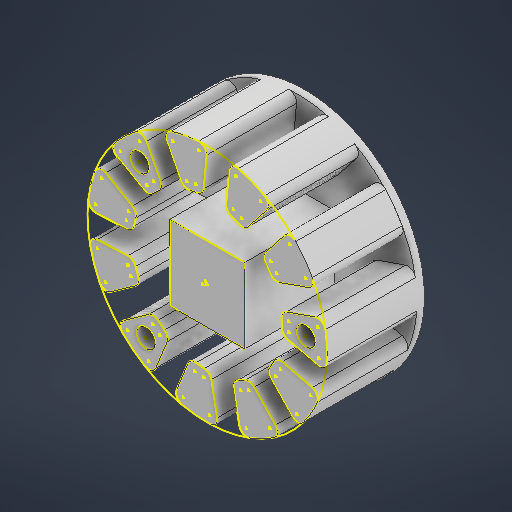
# Autodesk Inventor part: новая сиська 5-26
Saved by Autodesk Inventor 2025 (Build 290162000, 162)
## iProperties
Created: 2025-10-01
Part Number: новая сиська 5-26
Material: Типовые
Document SubType Name: Modeling
Designer: GameHD
Density: 1 g/cm^3
Appearance: По умолчанию
Author: GameHD
Autodesk Inventor part; units mm, degrees
ref_plane "YZ Plane" through (0, 0, 0) normal (1, 0, 0) x (0, 1, 0)
ref_plane "XZ Plane" through (0, 0, 0) normal (0, 1, 0) x (-1, 0, 0)
ref_plane "XY Plane" through (0, 0, 0) normal (0, 0, 1) x (1, 0, 0)
sketch "Эскиз1" plane through (0, 0, 0) normal (0, 0, 1) x (1, 0, 0)
  arc A0 (22.5563, 14.1182) -> (20.9448, 16.3602) centre (1.564, 0.7293) ccw
  arc A1 (20.9188, 19.4663) -> (20.9448, 16.3602) centre (22.8907, 17.9297) ccw
  line L0 (20.9188, 19.4663) -> (27.2495, 27.5902)
  arc A2 (31.0653, 27.7418) -> (27.2495, 27.5902) centre (29.2214, 26.0536) ccw
  arc A3 (36.5698, 20.0838) -> (31.0653, 27.7418) centre (1.564, 0.7293) ccw
  arc A4 (35.2101, 16.5153) -> (36.5698, 20.0838) centre (34.382, 18.8741) ccw
  line L1 (35.2101, 16.5153) -> (25.4922, 13.1036)
  arc A5 (22.5563, 14.1182) -> (25.4922, 13.1036) centre (24.6641, 15.4625) ccw
  line L2 (-22.3857, -11.7684) -> (-30.7753, -17.7426)
  arc A6 (-34.475, -16.7967) -> (-30.7753, -17.7426) centre (-32.2254, -15.7062) ccw
  arc A7 (-37.5597, -7.8842) -> (-34.475, -16.7967) centre (1.5191, 0.651) ccw
  arc A8 (-35.2362, -4.8536) -> (-37.5597, -7.8842) centre (-35.1172, -7.3508) ccw
  line L3 (-35.2362, -4.8536) -> (-24.9486, -4.3636)
  arc A9 (-22.4254, -6.1753) -> (-24.9486, -4.3636) centre (-24.8296, -6.8607) ccw
  arc A10 (-22.4254, -6.1753) -> (-21.5223, -8.7846) centre (1.5191, 0.651) ccw
  arc A11 (-22.3857, -11.7684) -> (-21.5223, -8.7846) centre (-23.8358, -9.732) ccw
  line L4 (-11.8764, -22.7208) -> (-15.7043, -32.2823)
  arc A12 (-19.3282, -33.4868) -> (-15.7043, -32.2823) centre (-18.0252, -31.3532) ccw
  arc A13 (-26.7415, -27.6569) -> (-19.3282, -33.4868) centre (1.5191, 0.651) ccw
  arc A14 (-26.4254, -23.8512) -> (-26.7415, -27.6569) centre (-24.9752, -25.8876) ccw
  line L5 (-26.4254, -23.8512) -> (-18.0358, -17.877)
  arc A15 (-14.9337, -18.037) -> (-18.0358, -17.877) centre (-16.5857, -19.9134) ccw
  arc A16 (-14.9337, -18.037) -> (-12.7633, -19.7438) centre (1.5191, 0.651) ccw
  arc A17 (-11.8764, -22.7208) -> (-12.7633, -19.7438) centre (-14.1973, -21.7916) ccw
  line L6 (-19.7085, 17.2364) -> (-28.6279, 22.386)
  arc A18 (-29.3044, 26.1444) -> (-28.6279, 22.386) centre (-27.3779, 24.5511) ccw
  arc A19 (-22.4788, 32.6526) -> (-29.3044, 26.1444) centre (1.5191, 0.651) ccw
  arc A20 (-18.7568, 31.7981) -> (-22.4788, 32.6526) centre (-20.9789, 30.6525) ccw
  line L7 (-18.7568, 31.7981) -> (-14.0374, 22.6437)
  arc A21 (-14.6373, 19.5959) -> (-14.0374, 22.6437) centre (-16.2595, 21.4982) ccw
  arc A22 (-14.6373, 19.5959) -> (-16.6356, 17.6905) centre (1.5191, 0.651) ccw
  arc A23 (-19.7085, 17.2364) -> (-16.6356, 17.6905) centre (-18.4585, 19.4014) ccw
  line L8 (26.5594, -9.282) -> (36.5684, -11.7101)
  arc A24 (38.2763, -15.1257) -> (36.5684, -11.7101) centre (35.979, -14.1397) ccw
  arc A25 (33.5608, -23.2933) -> (38.2763, -15.1257) centre (1.5191, 0.651) ccw
  arc A26 (29.7488, -23.522) -> (33.5608, -23.2933) centre (31.5582, -21.7968) ccw
  line L9 (29.7488, -23.522) -> (22.6415, -16.068)
  arc A27 (22.3584, -12.9747) -> (22.6415, -16.068) centre (24.4508, -14.3428) ccw
  arc A28 (22.3584, -12.9747) -> (23.739, -10.5835) centre (1.5191, 0.651) ccw
  arc A29 (26.5594, -9.282) -> (23.739, -10.5835) centre (25.97, -11.7115) ccw
  line L10 (27.9545, 5.8327) -> (37.6874, 9.2013)
  arc A30 (40.9708, 7.2513) -> (37.6874, 9.2013) centre (38.5051, 6.8388) ccw
  arc A31 (41.4196, -2.1692) -> (40.9708, 7.2513) centre (1.5191, 0.651) ccw
  arc A32 (38.3364, -4.4224) -> (41.4196, -2.1692) centre (38.9258, -1.9929) ccw
  line L11 (38.3364, -4.4224) -> (28.3274, -1.9943)
  arc A33 (26.4169, 0.4549) -> (28.3274, -1.9943) centre (28.9168, 0.4352) ccw
  arc A34 (26.4169, 0.4549) -> (26.2855, 3.2129) centre (1.5191, 0.651) ccw
  arc A35 (27.9545, 5.8327) -> (26.2855, 3.2129) centre (28.7722, 3.4702) ccw
  line L12 (-7.372, 26.08) -> (-12.0914, 35.2344)
  arc A36 (-10.6285, 38.7619) -> (-12.0914, 35.2344) centre (-9.8693, 36.3799) ccw
  arc A37 (-1.3678, 40.5467) -> (-10.6285, 38.7619) centre (1.5191, 0.651) ccw
  arc A38 (1.3013, 37.8156) -> (-1.3678, 40.5467) centre (-1.1874, 38.0532) ccw
  line L13 (1.3013, 37.8156) -> (0.3223, 27.5629)
  arc A39 (-1.8301, 25.3233) -> (0.3223, 27.5629) centre (-2.1664, 27.8006) ccw
  arc A40 (-1.8301, 25.3233) -> (-4.5414, 24.8007) centre (1.5191, 0.651) ccw
  arc A41 (-7.372, 26.08) -> (-4.5414, 24.8007) centre (-5.1499, 27.2256) ccw
  line L14 (2.8858, -26.2528) -> (4.835, -36.3659)
  arc A42 (2.4376, -39.3384) -> (4.835, -36.3659) centre (2.3802, -36.8391) ccw
  arc A43 (-6.9508, -38.4419) -> (2.4376, -39.3384) centre (1.5191, 0.651) ccw
  arc A44 (-8.7424, -35.0695) -> (-6.9508, -38.4419) centre (-6.4215, -35.9986) ccw
  line L15 (-8.7424, -35.0695) -> (-4.9145, -25.5079)
  arc A45 (-2.2183, -23.9654) -> (-4.9145, -25.5079) centre (-2.5936, -26.4371) ccw
  arc A46 (-2.2183, -23.9654) -> (0.5303, -24.2279) centre (1.5191, 0.651) ccw
  arc A47 (2.8858, -26.2528) -> (0.5303, -24.2279) centre (0.431, -26.7259) ccw
  line L16 (-25.3054, 3.127) -> (-35.593, 2.637)
  arc A48 (-38.194, 5.433) -> (-35.593, 2.637) centre (-35.712, 5.1341) ccw
  arc A49 (-35.9706, 14.5983) -> (-38.194, 5.433) centre (1.5191, 0.651) ccw
  arc A50 (-32.3775, 15.8916) -> (-35.9706, 14.5983) centre (-33.6275, 13.7266) ccw
  line L17 (-32.3775, 15.8916) -> (-23.458, 10.742)
  arc A51 (-22.3149, 7.8537) -> (-23.458, 10.742) centre (-24.708, 8.5769) ccw
  arc A52 (-22.3149, 7.8537) -> (-22.9659, 5.1704) centre (1.5191, 0.651) ccw
  arc A53 (-25.3054, 3.127) -> (-22.9659, 5.1704) centre (-25.4243, 5.6242) ccw
  line L18 (17.2148, -21.2437) -> (24.3215, -28.6969)
  arc A54 (23.9117, -32.4937) -> (24.3215, -28.6969) centre (22.5122, -30.4221) ccw
  arc A55 (15.529, -36.8153) -> (23.9117, -32.4937) centre (1.5191, 0.651) ccw
  arc A56 (12.1985, -34.9467) -> (15.529, -36.8153) centre (14.6534, -34.4736) ccw
  line L19 (12.1985, -34.9467) -> (10.2513, -24.8433)
  arc A57 (11.676, -22.0923) -> (10.2513, -24.8433) centre (12.7061, -24.3702) ccw
  arc A58 (11.676, -22.0923) -> (14.1352, -20.8156) centre (1.1306, 1.228) ccw
  arc A59 (17.2148, -21.2437) -> (14.1352, -20.8156) centre (15.4055, -22.9689) ccw
  line L20 (7.7874, 26.8501) -> (8.7664, 37.1028)
  arc A60 (11.9042, 39.2794) -> (8.7664, 37.1028) centre (11.2551, 36.8651) ccw
  arc A61 (20.6597, 35.7742) -> (11.9042, 39.2794) centre (1.5191, 0.651) ccw
  arc A62 (21.4285, 32.0336) -> (20.6597, 35.7742) centre (19.4634, 33.579) ccw
  line L21 (21.4285, 32.0336) -> (15.0619, 23.9378)
  arc A63 (12.0404, 23.2174) -> (15.0619, 23.9378) centre (13.0968, 25.4832) ccw
  arc A64 (12.0404, 23.2174) -> (9.477, 24.2436) centre (1.5191, 0.651) ccw
  arc A65 (7.7874, 26.8501) -> (9.477, 24.2436) centre (10.2761, 26.6125) ccw
  circle A66 centre (1.5191, 0.651) radius 50
  line L22 (19.1721, 10.843) -> (19.1721, -9.5409)
  line L23 (19.1721, -9.5409) -> (1.5191, -19.7329)
  line L24 (1.5191, -19.7329) -> (-16.1339, -9.5409)
  line L25 (-16.1339, -9.5409) -> (-16.1339, 10.843)
  line L26 (-16.1339, 10.843) -> (1.5191, 21.035)
  line L27 (1.5191, 21.035) -> (19.1721, 10.843)
  point P0 (0, 0)
  point P1 (1.5191, 0.651)
  dimension "d9" = 100
  constraints: 132 point on circle, 67 centre point, 56 end point
  measures "d9" diameter of A66
extrude "Выдавливание1" add sketch "Эскиз1" along normal blind 30 contours A0 A1 L0 A2 A3 A4 L1 A5 | L2 A6 A7 A8 L3 A9 A10 A11 | L4 A12 A13 A14 L5 A15 A16 A17 | L6 A18 A19 A20 L7 A21 A22 A23 | L8 A24 A25 A26 L9 A27 A28 A29 | L10 A30 A31 A32 L11 A33 A34 A35 | L12 A36 A37 A38 L13 A39 A40 A41 | L14 A42 A43 A44 L15 A45 A46 A47 | L16 A48 A49 A50 L17 A51 A52 A53 | L18 A54 A55 A56 L19 A57 A58 A59 | L20 A60 A61 A62 L21 A63 A64 A65 | L22 L23 L24 L25 L26 L27
sketch "Эскиз2" plane through (0, 0, 0) normal (0, 0, -1) x (-1, 0, 0)
  line L0 (-19.1721, 10.843) -> (-1.5191, 21.035) projected
  line L1 (-19.1721, -9.5409) -> (-19.1721, 10.843) projected
  line L2 (-1.5191, -19.7329) -> (-19.1721, -9.5409) projected
  line L3 (16.1339, -9.5409) -> (-1.5191, -19.7329) projected
  line L4 (16.1339, 10.843) -> (16.1339, -9.5409) projected
  line L5 (-1.5191, 21.035) -> (16.1339, 10.843) projected
  arc A0 (-11.9042, 39.2794) -> (-20.6597, 35.7742) centre (-1.5191, 0.651) ccw projected
  circle A1 centre (-1.5191, 0.651) radius 40
  point P0 (0, 0)
  dimension "d2" = 80
  constraints: 1 centre point, 1 coincident
  measures "d2" diameter of A1
extrude "Выдавливание2" add sketch "Эскиз2" along normal blind 2.5 contours L0 L5 L4 L3 L2 L1 | A1 A0
sketch "Эскиз3" plane through (0, 0, 30) normal (0, 0, 1) x (1, 0, 0)
  line L0 (19.1721, 10.843) -> (1.5191, 21.035) projected
  line L1 (1.5191, 21.035) -> (-16.1339, 10.843) projected
  line L2 (-16.1339, 10.843) -> (-16.1339, -9.5409) projected
  line L3 (-16.1339, -9.5409) -> (1.5191, -19.7329) projected
  line L4 (1.5191, -19.7329) -> (19.1721, -9.5409) projected
  line L5 (19.1721, -9.5409) -> (19.1721, 10.843) projected
  arc A0 (-22.4788, 32.6526) -> (-29.3044, 26.1444) centre (1.5191, 0.651) ccw projected
  line L6 (14.0191, -11.849) -> (-10.9809, -11.849)
  line L7 (-10.9809, -11.849) -> (-10.9809, 13.151)
  line L8 (-10.9809, 13.151) -> (14.0191, 13.151)
  line L9 (14.0191, 13.151) -> (14.0191, -11.849)
  line L10 (14.0191, -11.849) -> (-10.9809, 13.151) construction
  line L11 (-10.9809, -11.849) -> (14.0191, 13.151) construction
  point P0 (0, 0)
  dimension "d5" = 25
  dimension "d6" = 25
  constraints: 12 end point, 2 midpoint, 2 parallel, 1 horizontal, 1 perpendicular
  measures "d5" distance of L7.end L8.end
  measures "d6" distance of L6.end L7.end
extrude "Выдавливание3" cut sketch "Эскиз3" against normal up to surface (30 mm away)
sketch "Эскиз6" plane through (0, 0, 30) normal (0, 0, 1) x (1, 0, 0)
  circle A0 centre (34.4254, 2.0527) radius 3.1 projected
  circle A1 centre (-21.0893, 24.6021) radius 3.1 projected
  circle A2 centre (-18.9706, -25.1358) radius 3.1 projected
  point P0 (0, 0)
extrude "Выдавливание5" cut sketch "Эскиз6" against normal through all
sketch "Эскиз7" plane through (0, 0, 30) normal (0, 0, 1) x (1, 0, 0)
  line L0 (-10.9809, -11.849) -> (-10.9809, 13.151) projected
  line L1 (-10.9809, 13.151) -> (14.0191, 13.151) projected
  line L2 (14.0191, 13.151) -> (14.0191, -11.849) projected
  line L3 (14.0191, -11.849) -> (-10.9809, -11.849) projected
  arc A0 (21.4285, 32.0336) -> (20.6597, 35.7742) centre (19.4634, 33.579) ccw projected
  line L4 (15.0619, 23.9378) -> (21.4285, 32.0336) projected
  arc A1 (12.0404, 23.2174) -> (15.0619, 23.9378) centre (13.0968, 25.4832) ccw projected
  arc A2 (12.0404, 23.2174) -> (9.477, 24.2436) centre (1.5191, 0.651) ccw projected
  arc A3 (7.7874, 26.8501) -> (9.477, 24.2436) centre (10.2761, 26.6125) ccw projected
  line L5 (8.7664, 37.1028) -> (7.7874, 26.8501) projected
  arc A4 (11.9042, 39.2794) -> (8.7664, 37.1028) centre (11.2551, 36.8651) ccw projected
  arc A5 (11.9042, 39.2794) -> (-1.3678, 40.5467) centre (1.5191, 0.651) ccw projected
  arc A6 (1.3013, 37.8156) -> (-1.3678, 40.5467) centre (-1.1874, 38.0532) ccw projected
  line L6 (0.3223, 27.5629) -> (1.3013, 37.8156) projected
  arc A7 (-1.8301, 25.3233) -> (0.3223, 27.5629) centre (-2.1664, 27.8006) ccw projected
  arc A8 (-1.8301, 25.3233) -> (-4.5414, 24.8007) centre (1.5191, 0.651) ccw projected
  arc A9 (-7.372, 26.08) -> (-4.5414, 24.8007) centre (-5.1499, 27.2256) ccw projected
  line L7 (-12.0914, 35.2344) -> (-7.372, 26.08) projected
  arc A10 (-10.6285, 38.7619) -> (-12.0914, 35.2344) centre (-9.8693, 36.3799) ccw projected
  arc A11 (-10.6285, 38.7619) -> (-22.4788, 32.6526) centre (1.5191, 0.651) ccw projected
  arc A12 (-18.7568, 31.7981) -> (-22.4788, 32.6526) centre (-20.9789, 30.6525) ccw projected
  line L8 (-14.0374, 22.6437) -> (-18.7568, 31.7981) projected
  arc A13 (-14.6373, 19.5959) -> (-14.0374, 22.6437) centre (-16.2595, 21.4982) ccw projected
  arc A14 (-14.6373, 19.5959) -> (-16.6356, 17.6905) centre (1.5191, 0.651) ccw projected
  arc A15 (-19.7085, 17.2364) -> (-16.6356, 17.6905) centre (-18.4585, 19.4014) ccw projected
  line L9 (-28.6279, 22.386) -> (-19.7085, 17.2364) projected
  arc A16 (-29.3044, 26.1444) -> (-28.6279, 22.386) centre (-27.3779, 24.5511) ccw projected
  arc A17 (-29.3044, 26.1444) -> (-35.9706, 14.5983) centre (1.5191, 0.651) ccw projected
  arc A18 (-32.3775, 15.8916) -> (-35.9706, 14.5983) centre (-33.6275, 13.7266) ccw projected
  line L10 (-23.458, 10.742) -> (-32.3775, 15.8916) projected
  arc A19 (-22.3149, 7.8537) -> (-23.458, 10.742) centre (-24.708, 8.5769) ccw projected
  arc A20 (-22.3149, 7.8537) -> (-22.9659, 5.1704) centre (1.5191, 0.651) ccw projected
  arc A21 (-25.3054, 3.127) -> (-22.9659, 5.1704) centre (-25.4243, 5.6242) ccw projected
  line L11 (-35.593, 2.637) -> (-25.3054, 3.127) projected
  arc A22 (-38.194, 5.433) -> (-35.593, 2.637) centre (-35.712, 5.1341) ccw projected
  arc A23 (-38.194, 5.433) -> (-37.5597, -7.8842) centre (1.5191, 0.651) ccw projected
  arc A24 (-35.2362, -4.8536) -> (-37.5597, -7.8842) centre (-35.1172, -7.3508) ccw projected
  line L12 (-24.9486, -4.3636) -> (-35.2362, -4.8536) projected
  arc A25 (-22.4254, -6.1753) -> (-24.9486, -4.3636) centre (-24.8296, -6.8607) ccw projected
  arc A26 (-22.4254, -6.1753) -> (-21.5223, -8.7846) centre (1.5191, 0.651) ccw projected
  arc A27 (-22.3857, -11.7684) -> (-21.5223, -8.7846) centre (-23.8358, -9.732) ccw projected
  line L13 (-30.7753, -17.7426) -> (-22.3857, -11.7684) projected
  arc A28 (-34.475, -16.7967) -> (-30.7753, -17.7426) centre (-32.2254, -15.7062) ccw projected
  arc A29 (-34.475, -16.7967) -> (-26.7415, -27.6569) centre (1.5191, 0.651) ccw projected
  arc A30 (-26.4254, -23.8512) -> (-26.7415, -27.6569) centre (-24.9752, -25.8876) ccw projected
  line L14 (-18.0358, -17.877) -> (-26.4254, -23.8512) projected
  arc A31 (-14.9337, -18.037) -> (-18.0358, -17.877) centre (-16.5857, -19.9134) ccw projected
  arc A32 (-14.9337, -18.037) -> (-12.7633, -19.7438) centre (1.5191, 0.651) ccw projected
  arc A33 (-11.8764, -22.7208) -> (-12.7633, -19.7438) centre (-14.1973, -21.7916) ccw projected
  line L15 (-15.7043, -32.2823) -> (-11.8764, -22.7208) projected
  arc A34 (-19.3282, -33.4868) -> (-15.7043, -32.2823) centre (-18.0252, -31.3532) ccw projected
  arc A35 (-19.3282, -33.4868) -> (-6.9508, -38.4419) centre (1.5191, 0.651) ccw projected
  arc A36 (-8.7424, -35.0695) -> (-6.9508, -38.4419) centre (-6.4215, -35.9986) ccw projected
  line L16 (-4.9145, -25.5079) -> (-8.7424, -35.0695) projected
  arc A37 (-2.2183, -23.9654) -> (-4.9145, -25.5079) centre (-2.5936, -26.4371) ccw projected
  arc A38 (-2.2183, -23.9654) -> (0.5303, -24.2279) centre (1.5191, 0.651) ccw projected
  arc A39 (2.8858, -26.2528) -> (0.5303, -24.2279) centre (0.431, -26.7259) ccw projected
  line L17 (4.835, -36.3659) -> (2.8858, -26.2528) projected
  arc A40 (2.4376, -39.3384) -> (4.835, -36.3659) centre (2.3802, -36.8391) ccw projected
  arc A41 (2.4376, -39.3384) -> (15.529, -36.8153) centre (1.5191, 0.651) ccw projected
  arc A42 (12.1985, -34.9467) -> (15.529, -36.8153) centre (14.6534, -34.4736) ccw projected
  line L18 (10.2513, -24.8433) -> (12.1985, -34.9467) projected
  arc A43 (11.676, -22.0923) -> (10.2513, -24.8433) centre (12.7061, -24.3702) ccw projected
  arc A44 (11.676, -22.0923) -> (14.1352, -20.8156) centre (1.1306, 1.228) ccw projected
  arc A45 (17.2148, -21.2437) -> (14.1352, -20.8156) centre (15.4055, -22.9689) ccw projected
  line L19 (24.3215, -28.6969) -> (17.2148, -21.2437) projected
  arc A46 (23.9117, -32.4937) -> (24.3215, -28.6969) centre (22.5122, -30.4221) ccw projected
  arc A47 (23.9117, -32.4937) -> (33.5608, -23.2933) centre (1.5191, 0.651) ccw projected
  arc A48 (29.7488, -23.522) -> (33.5608, -23.2933) centre (31.5582, -21.7968) ccw projected
  line L20 (22.6415, -16.068) -> (29.7488, -23.522) projected
  arc A49 (22.3584, -12.9747) -> (22.6415, -16.068) centre (24.4508, -14.3428) ccw projected
  arc A50 (22.3584, -12.9747) -> (23.739, -10.5835) centre (1.5191, 0.651) ccw projected
  arc A51 (26.5594, -9.282) -> (23.739, -10.5835) centre (25.97, -11.7115) ccw projected
  line L21 (36.5684, -11.7101) -> (26.5594, -9.282) projected
  arc A52 (38.2763, -15.1257) -> (36.5684, -11.7101) centre (35.979, -14.1397) ccw projected
  arc A53 (38.2763, -15.1257) -> (41.4196, -2.1692) centre (1.5191, 0.651) ccw projected
  arc A54 (38.3364, -4.4224) -> (41.4196, -2.1692) centre (38.9258, -1.9929) ccw projected
  line L22 (28.3274, -1.9943) -> (38.3364, -4.4224) projected
  arc A55 (26.4169, 0.4549) -> (28.3274, -1.9943) centre (28.9168, 0.4352) ccw projected
  arc A56 (26.4169, 0.4549) -> (26.2855, 3.2129) centre (1.5191, 0.651) ccw projected
  arc A57 (27.9545, 5.8327) -> (26.2855, 3.2129) centre (28.7722, 3.4702) ccw projected
  line L23 (37.6874, 9.2013) -> (27.9545, 5.8327) projected
  arc A58 (40.9708, 7.2513) -> (37.6874, 9.2013) centre (38.5051, 6.8388) ccw projected
  arc A59 (40.9708, 7.2513) -> (36.8048, 19.4902) centre (1.5191, 0.651) ccw projected
  arc A60 (35.2101, 16.5153) -> (36.8048, 19.4902) centre (34.382, 18.8741) ccw projected
  line L24 (25.4922, 13.1036) -> (35.2101, 16.5153) projected
  arc A61 (22.5563, 14.1182) -> (25.4922, 13.1036) centre (24.6641, 15.4625) ccw projected
  arc A62 (22.5563, 14.1182) -> (20.9448, 16.3602) centre (1.564, 0.7293) ccw projected
  arc A63 (20.9188, 19.4663) -> (20.9448, 16.3602) centre (22.8907, 17.9297) ccw projected
  line L25 (27.2495, 27.5902) -> (20.9188, 19.4663) projected
  arc A64 (30.5432, 28.1756) -> (27.2495, 27.5902) centre (29.2214, 26.0536) ccw projected
  arc A65 (30.5432, 28.1756) -> (20.6597, 35.7742) centre (1.5191, 0.651) ccw projected
  arc A66 (12.0404, 23.2174) -> (9.477, 24.2436) centre (1.5191, 0.651) ccw projected
  arc A67 (12.0404, 23.2174) -> (15.0619, 23.9378) centre (13.0968, 25.4832) ccw projected
  line L26 (15.0619, 23.9378) -> (21.4285, 32.0336) projected
  arc A68 (21.4285, 32.0336) -> (20.6597, 35.7742) centre (19.4634, 33.579) ccw projected
  arc A69 (20.6597, 35.7742) -> (11.9042, 39.2794) centre (1.5191, 0.651) ccw projected
  arc A70 (11.9042, 39.2794) -> (8.7664, 37.1028) centre (11.2551, 36.8651) ccw projected
  line L27 (8.7664, 37.1028) -> (7.7874, 26.8501) projected
  arc A71 (7.7874, 26.8501) -> (9.477, 24.2436) centre (10.2761, 26.6125) ccw projected
  line L28 (0.3223, 27.5629) -> (1.3013, 37.8156) projected
  arc A72 (1.3013, 37.8156) -> (-1.3678, 40.5467) centre (-1.1874, 38.0532) ccw projected
  arc A73 (-1.3678, 40.5467) -> (-10.6285, 38.7619) centre (1.5191, 0.651) ccw projected
  arc A74 (-10.6285, 38.7619) -> (-12.0914, 35.2344) centre (-9.8693, 36.3799) ccw projected
  line L29 (-12.0914, 35.2344) -> (-7.372, 26.08) projected
  arc A75 (-7.372, 26.08) -> (-4.5414, 24.8007) centre (-5.1499, 27.2256) ccw projected
  arc A76 (-1.8301, 25.3233) -> (-4.5414, 24.8007) centre (1.5191, 0.651) ccw projected
  arc A77 (-1.8301, 25.3233) -> (0.3223, 27.5629) centre (-2.1664, 27.8006) ccw projected
  circle A78 centre (-21.0893, 24.6021) radius 3.1 projected
  arc A79 (-14.6373, 19.5959) -> (-16.6356, 17.6905) centre (1.5191, 0.651) ccw projected
  arc A80 (-14.6373, 19.5959) -> (-14.0374, 22.6437) centre (-16.2595, 21.4982) ccw projected
  line L30 (-14.0374, 22.6437) -> (-18.7568, 31.7981) projected
  arc A81 (-18.7568, 31.7981) -> (-22.4788, 32.6526) centre (-20.9789, 30.6525) ccw projected
  arc A82 (-22.4788, 32.6526) -> (-29.3044, 26.1444) centre (1.5191, 0.651) ccw projected
  arc A83 (-29.3044, 26.1444) -> (-28.6279, 22.386) centre (-27.3779, 24.5511) ccw projected
  line L31 (-28.6279, 22.386) -> (-19.7085, 17.2364) projected
  arc A84 (-19.7085, 17.2364) -> (-16.6356, 17.6905) centre (-18.4585, 19.4014) ccw projected
  arc A85 (-35.9706, 14.5983) -> (-38.194, 5.433) centre (1.5191, 0.651) ccw projected
  arc A86 (-38.194, 5.433) -> (-35.593, 2.637) centre (-35.712, 5.1341) ccw projected
  line L32 (-35.593, 2.637) -> (-25.3054, 3.127) projected
  arc A87 (-25.3054, 3.127) -> (-22.9659, 5.1704) centre (-25.4243, 5.6242) ccw projected
  arc A88 (-22.3149, 7.8537) -> (-22.9659, 5.1704) centre (1.5191, 0.651) ccw projected
  arc A89 (-22.3149, 7.8537) -> (-23.458, 10.742) centre (-24.708, 8.5769) ccw projected
  line L33 (-23.458, 10.742) -> (-32.3775, 15.8916) projected
  arc A90 (-32.3775, 15.8916) -> (-35.9706, 14.5983) centre (-33.6275, 13.7266) ccw projected
  arc A91 (-37.5597, -7.8842) -> (-34.475, -16.7967) centre (1.5191, 0.651) ccw projected
  arc A92 (-34.475, -16.7967) -> (-30.7753, -17.7426) centre (-32.2254, -15.7062) ccw projected
  line L34 (-30.7753, -17.7426) -> (-22.3857, -11.7684) projected
  arc A93 (-22.3857, -11.7684) -> (-21.5223, -8.7846) centre (-23.8358, -9.732) ccw projected
  arc A94 (-22.4254, -6.1753) -> (-21.5223, -8.7846) centre (1.5191, 0.651) ccw projected
  arc A95 (-22.4254, -6.1753) -> (-24.9486, -4.3636) centre (-24.8296, -6.8607) ccw projected
  line L35 (-24.9486, -4.3636) -> (-35.2362, -4.8536) projected
  arc A96 (-35.2362, -4.8536) -> (-37.5597, -7.8842) centre (-35.1172, -7.3508) ccw projected
  arc A97 (-6.9508, -38.4419) -> (2.4376, -39.3384) centre (1.5191, 0.651) ccw projected
  arc A98 (2.4376, -39.3384) -> (4.835, -36.3659) centre (2.3802, -36.8391) ccw projected
  line L36 (4.835, -36.3659) -> (2.8858, -26.2528) projected
  arc A99 (2.8858, -26.2528) -> (0.5303, -24.2279) centre (0.431, -26.7259) ccw projected
  arc A100 (-2.2183, -23.9654) -> (0.5303, -24.2279) centre (1.5191, 0.651) ccw projected
  arc A101 (-2.2183, -23.9654) -> (-4.9145, -25.5079) centre (-2.5936, -26.4371) ccw projected
  line L37 (-4.9145, -25.5079) -> (-8.7424, -35.0695) projected
  arc A102 (-8.7424, -35.0695) -> (-6.9508, -38.4419) centre (-6.4215, -35.9986) ccw projected
  arc A103 (15.529, -36.8153) -> (23.9117, -32.4937) centre (1.5191, 0.651) ccw projected
  arc A104 (23.9117, -32.4937) -> (24.3215, -28.6969) centre (22.5122, -30.4221) ccw projected
  line L38 (24.3215, -28.6969) -> (17.2148, -21.2437) projected
  arc A105 (17.2148, -21.2437) -> (14.1352, -20.8156) centre (15.4055, -22.9689) ccw projected
  arc A106 (11.676, -22.0923) -> (14.1352, -20.8156) centre (1.1306, 1.228) ccw projected
  arc A107 (11.676, -22.0923) -> (10.2513, -24.8433) centre (12.7061, -24.3702) ccw projected
  line L39 (10.2513, -24.8433) -> (12.1985, -34.9467) projected
  arc A108 (12.1985, -34.9467) -> (15.529, -36.8153) centre (14.6534, -34.4736) ccw projected
  circle A109 centre (-18.9706, -25.1358) radius 3.1 projected
  arc A110 (-26.7415, -27.6569) -> (-19.3282, -33.4868) centre (1.5191, 0.651) ccw projected
  arc A111 (-19.3282, -33.4868) -> (-15.7043, -32.2823) centre (-18.0252, -31.3532) ccw projected
  line L40 (-15.7043, -32.2823) -> (-11.8764, -22.7208) projected
  arc A112 (-11.8764, -22.7208) -> (-12.7633, -19.7438) centre (-14.1973, -21.7916) ccw projected
  arc A113 (-14.9337, -18.037) -> (-12.7633, -19.7438) centre (1.5191, 0.651) ccw projected
  arc A114 (-14.9337, -18.037) -> (-18.0358, -17.877) centre (-16.5857, -19.9134) ccw projected
  line L41 (-18.0358, -17.877) -> (-26.4254, -23.8512) projected
  arc A115 (-26.4254, -23.8512) -> (-26.7415, -27.6569) centre (-24.9752, -25.8876) ccw projected
  arc A116 (22.3584, -12.9747) -> (23.739, -10.5835) centre (1.5191, 0.651) ccw projected
  arc A117 (22.3584, -12.9747) -> (22.6415, -16.068) centre (24.4508, -14.3428) ccw projected
  line L42 (22.6415, -16.068) -> (29.7488, -23.522) projected
  arc A118 (29.7488, -23.522) -> (33.5608, -23.2933) centre (31.5582, -21.7968) ccw projected
  arc A119 (33.5608, -23.2933) -> (38.2763, -15.1257) centre (1.5191, 0.651) ccw projected
  arc A120 (38.2763, -15.1257) -> (36.5684, -11.7101) centre (35.979, -14.1397) ccw projected
  line L43 (36.5684, -11.7101) -> (26.5594, -9.282) projected
  arc A121 (26.5594, -9.282) -> (23.739, -10.5835) centre (25.97, -11.7115) ccw projected
  circle A122 centre (34.4254, 2.0527) radius 3.1 projected
  line L44 (28.3274, -1.9943) -> (38.3364, -4.4224) projected
  arc A123 (38.3364, -4.4224) -> (41.4196, -2.1692) centre (38.9258, -1.9929) ccw projected
  arc A124 (41.4196, -2.1692) -> (40.9708, 7.2513) centre (1.5191, 0.651) ccw projected
  arc A125 (40.9708, 7.2513) -> (37.6874, 9.2013) centre (38.5051, 6.8388) ccw projected
  line L45 (37.6874, 9.2013) -> (27.9545, 5.8327) projected
  arc A126 (27.9545, 5.8327) -> (26.2855, 3.2129) centre (28.7722, 3.4702) ccw projected
  arc A127 (26.4169, 0.4549) -> (26.2855, 3.2129) centre (1.5191, 0.651) ccw projected
  arc A128 (26.4169, 0.4549) -> (28.3274, -1.9943) centre (28.9168, 0.4352) ccw projected
  point P0 (0, 0)
